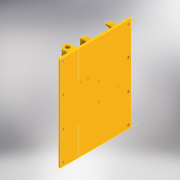
# Autodesk Inventor part: Carcasa
Saved by Autodesk Inventor 2021 (Build 250183000, 183)
## iProperties
Created: 2024-02-25
Part Number: Carcasa
Material: PLA
Document SubType Name: Modeling
Designer: Martin
Density: 1.27 g/cm^3
Appearance: PLA
Mass: 404.193 g
Surface Area: 1591.38 cm^2
Volume: 318.262 cm^3
Author: Martin
Autodesk Inventor part; units mm, degrees
ref_plane "YZ Plane" through (0, 0, 0) normal (1, 0, 0) x (0, 1, 0)
ref_plane "XZ Plane" through (0, 0, 0) normal (0, 1, 0) x (-1, 0, 0)
ref_plane "XY Plane" through (0, 0, 0) normal (0, 0, 1) x (1, 0, 0)
sketch "Sketch1" plane through (0, 0, 0) normal (0, 1, 0) x (-1, 0, 0)
  circle A0 centre (14, 22.0693) radius 4.1
  line L0 (0, 9.3293) -> (0, 34.8093) projected
  circle A1 centre (14, 22.0693) radius 9.1
  line L1 (14, 12.9693) -> (0, 12.9693)
  line L2 (14, 31.1693) -> (0, 31.1693)
  dimension "d0" = 8.2
  dimension "d7" = 14
  dimension "d20" = 5
  constraints: 4 end point, 2 centre point, 2 point on circle, 2 point on line, 1 parallel, 1 perpendicular
  measures "d0" diameter of A0
  measures "d7" distance from line of L0 A0.centre
  measures "d20" radial gap between concentric circles of A0 A1
extrude "Extrusion1" add sketch "Sketch1" along normal blind 60
sketch "Sketch3" plane through (0, 0, 0) normal (1, 0, 0) x (0, 1, 0)
  line L0 (0, 8.1261) -> (0, 35.9865) projected
  line L1 (0, 35.9865) -> (60, 35.9865) projected
  line L2 (60, 8.1261) -> (60, 35.9865) projected
  line L3 (0, 8.1261) -> (60, 8.1261) projected
  line L4 (0, 12.9691) -> (60, 12.9691)
  line L5 (60, 12.9691) -> (60, -77.0309)
  line L6 (60, -77.0309) -> (0, -77.0309)
  line L7 (8, -77.0309) -> (8, 12.9691)
  line L8 (12, -73.0309) -> (64, -73.0309)
  line L9 (56, -18.0309) -> (56, -14.0309)
  line L10 (-3, -73.0309) -> (37, -73.0309)
  line L11 (45, -75.0309) -> (45, -18.0309)
  line L12 (45, -18.0309) -> (12, -18.0309)
  line L13 (8, -14.0309) -> (49, -14.0309)
  line L14 (49.0192, -13.1359) -> (49.0192, -77.0309)
  line L15 (41.0192, -77.0309) -> (7, -77.0309)
  line L16 (8, -77.0309) -> (8, -14.0309)
  line L17 (12, -18.0309) -> (12, -24.0309)
  line L18 (12, -24.0309) -> (8, -24.0309)
  line L19 (-3, -73.0309) -> (0, -73.0309)
  line L20 (60, 17.9693) -> (0, 17.9693) projected
  line L21 (0, 12.9693) -> (60, 12.9693) projected
  line L22 (0, 12.9693) -> (0, 31.1693) projected
  line L23 (8, -73.0309) -> (12, -73.0309)
  line L24 (12, -73.0309) -> (12, -67.0309)
  line L25 (12, -67.0309) -> (8, -67.0309)
  line L26 (0, -67.0309) -> (0, -73.0309)
  line L27 (41, -14.0309) -> (0, -14.0309)
  line L28 (8, -14.0309) -> (8, -77.0309)
  line L29 (0, -77.0309) -> (41, -77.0309)
  line L30 (49, -77.0309) -> (49, -14.0309)
  line L31 (4, -73.0309) -> (37, -73.0309)
  line L32 (45, -73.0309) -> (45, -18.0309)
  line L33 (45, -18.0309) -> (12, -18.0309)
  line L34 (12, -18.0309) -> (12, -24.0309)
  line L35 (4, -67.0309) -> (4, -73.0309)
  line L36 (0, -77.0309) -> (0, 12.9691)
  line L37 (45, -75.0309) -> (12, -75.0309)
  line L38 (12, -75.0309) -> (12, -73.0309)
  line L39 (41.0192, -79.0309) -> (7, -79.0309)
  line L40 (8, -77.0309) -> (8, -79.0309)
  line L41 (41.0192, -79.0309) -> (49, -79.0309)
  line L42 (49, -79.0309) -> (49, -77.0309)
  line L43 (8, -67.0309) -> (6, -67.0309)
  line L44 (6, -67.0309) -> (6, -79.0309)
  line L45 (6, -79.0309) -> (8, -79.0309)
  line L46 (8, -14.0309) -> (6, -14.0309)
  line L47 (6, -24.0309) -> (6, -14.0309)
  line L48 (6, -24.0309) -> (8, -24.0309)
  line L49 (10, -24.0309) -> (10, -18.0309)
  line L50 (10, -18.0309) -> (12, -18.0309)
  line L51 (4, -73.0309) -> (4, -79.0309)
  line L52 (4, -79.0309) -> (6, -79.0309)
  line L53 (10, -67.0309) -> (10, -75.0309)
  line L54 (10, -75.0309) -> (12, -75.0309)
  line L55 (4, -67.0309) -> (6, -67.0309)
  line L56 (10, -75.0309) -> (8, -75.0309)
  point P0 (0, 0)
  point P1 (4, 104.056)
  point P2 (0, -73.0309)
  point P3 (49.0192, -73.0309)
  point P4 (49.0192, -77.0309)
  point P5 (8, -14.0309)
  point P6 (8, -24.0309)
  point P7 (45, -73.0309)
  point P8 (8, 8.1261)
  point P9 (0, -14.0309)
  point P10 (8, -73.0309)
  point P11 (8, -77.0309)
  point P12 (8, -67.0309)
  point P13 (12, -73.0309)
  point P14 (49, -73.0309)
  point P15 (0, -73.0309)
  point P16 (8, -77.0309)
  point P17 (6, -77.0309)
  dimension "d9" = 60
  dimension "d11" = 4
  dimension "d12" = 33
  dimension "d13" = 57
  dimension "d14" = 4
  dimension "d15" = 6
  dimension "d21" = 4
  dimension "d22" = 4
  dimension "d23" = 6
  dimension "d100" = 2
  dimension "d101" = 2
  constraints: 100 end point, 19 perpendicular, 13 parallel, 9 point on line, 8 horizontal, 5 vertical, 2 midpoint
  measures "d9" distance of L6.end L5.end
  measures "d11" distance between parallel lines of L6 L8
  measures "d12" distance of L12.end L11.end
  measures "d13" distance of L11.end L11.start
  measures "d14" distance between parallel lines of L12 L13
  measures "d15" distance of L12.end L17.end
  measures "d21" distance between parallel lines of L16 L17
  measures "d22" distance of L25.end L24.end
  measures "d23" distance of L35.end L35.start
  measures "d100" distance between parallel lines of L15 L39
  measures "d101" distance of L25.end L43.end
extrude "Extrusion2" add sketch "Sketch3" against normal blind 4 contours L0 L4 L7 L3 | L3 L7 L27 L36 | L7 L4 L2 L3 | L3 L5 L8 L30 L13 L7 | L27 L47 L48 L7 L43 L55 L35 L10 L26 L36 | L13 L30 L8 L11 L12 L50 L49 L18 L7 | L7 L48 L47 L27 | L5 L6 L14 L8 | L18 L17 L12 L11 L8 L24 L25 L7 | L10 L51 L6 L36 | L14 L6 L30 L8 | L25 L53 L10 L7 | L7 L10 L44 L43 | L49 L50 L17 L18 | L35 L55 L44 L10 | L10 L44 L6 L51 | L30 L6 L7 L56 L54 L37 L11 L8 | L10 L53 L56 L7 | L7 L6 L44 L10 | L25 L24 L10 L53 | L11 L37 L38 L8 | L10 L38 L54 L53
extrude "Extrusion3" add sketch "Sketch3" against normal blind 24 contours L13 L30 L8 L11 L12 L50 L49 L18 L7 | L7 L48 L47 L27 | L25 L53 L10 L7 | L7 L10 L44 L43 | L30 L6 L7 L56 L54 L37 L11 L8 | L10 L53 L56 L7 | L7 L6 L44 L10
sketch "Sketch5" plane through (0, 60, -77.0309) normal (0, 0, -1) x (-1, 0, 0)
  line L0 (0, -60) -> (14, -60) projected
  line L1 (14, -60) -> (14, 0) projected
  line L2 (0, 0) -> (14, 0) projected
  line L3 (0, -60) -> (0, 0) projected
  line L4 (4, -54) -> (4, -60) projected
  line L5 (0, 0) -> (4, 0) projected
  line L6 (0, -60) -> (0, 0) projected
  line L7 (0, -60) -> (4, -60) projected
  line L8 (24, -11) -> (24, -54) projected
  line L9 (0, 0) -> (4, 0)
  line L10 (4, 0) -> (4, -60)
  line L11 (4, -60) -> (0, -60)
  line L12 (0, -60) -> (0, 0)
  line L13 (4, 0) -> (4, -11) projected
  line L14 (4, -11) -> (24, -11) projected
  line L15 (4, -54) -> (24, -54) projected
  point P0 (4, -10.9808)
  constraints: 8 end point, 2 parallel, 1 horizontal, 1 perpendicular, 1 point on line
extrude "Extrusion4" add sketch "Sketch5" along normal blind 20 contours L3 L2 L10 L4 L0
sketch "Sketch6" plane through (-14, 0, 31.1693) normal (0, 0, 1) x (1, 0, 0)
  line L0 (10, 0) -> (10, 60) projected
  line L1 (0, 0) -> (14, 0) projected
  line L2 (14, 0) -> (14, 60) projected
  line L3 (0, 60) -> (14, 60) projected
  line L4 (0, 0) -> (0, 60) projected
extrude "Extrusion5" add sketch "Sketch6" along normal blind 20 contours L0 L3 L2 L1
sketch "Sketch8" plane through (-4, 0, 0) normal (-1, 0, 0) x (0, 0, 1)
  line L0 (31.1693, 0) -> (51.1693, 0) projected
  line L1 (31.1693, 0) -> (31.1693, 60) projected
  line L2 (31.1693, 0) -> (51.1693, 0) projected
  line L3 (51.1693, 60) -> (51.1693, 0) projected
  line L4 (31.1693, 60) -> (51.1693, 60) projected
  line L5 (51.1693, 60) -> (51.1693, 0) projected
  line L6 (-77.0309, 49) -> (-14.0309, 49) projected
  line L7 (-14.0309, 49) -> (-14.0309, 6) projected
  line L8 (-24.0309, 6) -> (-24.0309, 10) projected
  line L9 (-18.0309, 10) -> (-18.0309, 45) projected
  line L10 (-18.0309, 45) -> (-75.0309, 45) projected
  line L11 (-67.0309, 10) -> (-67.0309, 6) projected
  line L12 (-77.0309, 49) -> (-77.0309, 6) projected
  line L13 (12.9691, 60) -> (-97.0309, 60) projected
  line L14 (-97.0309, 0) -> (-97.0309, 60) projected
  line L15 (12.9691, 0) -> (-97.0309, 0) projected
  line L16 (12.9691, 0) -> (12.9691, 60) projected
  line L17 (-75.0309, 45) -> (-75.0309, 10) projected
  line L18 (-14.0309, 6) -> (-24.0309, 6) projected
  line L19 (-24.0309, 10) -> (-18.0309, 10) projected
  line L20 (-75.0309, 10) -> (-67.0309, 10) projected
  line L21 (-67.0309, 6) -> (-77.0309, 6) projected
  point P0 (0, 0)
  point P1 (45.1693, 8)
  point P2 (-91.0309, 8)
  point P3 (-97.0309, 90)
  dimension "d34" = 8
  dimension "d92" = 6
  dimension "d93" = 6
  dimension "d94" = 8
  measures "d34" distance from line of L0 point (45.169, 8)
  measures "d92" distance from line of L3 point (45.169, 8)
  measures "d93" distance from line of L14 point (-91.031, 8)
  measures "d94" distance from line of L15 point (-91.031, 8)
hole "Hole1" at (-4, 8, 45.1693) at (-4, 8, -91.0309) direction (1, 0, 0) diameter 4.134 depth 14.2 tip angle 118 thread size "M5x0.8" class "6H" standard "ISO Metric profile"
sketch "Sketch9" plane through (-4, 0, 0) normal (-1, 0, 0) x (0, 0, 1)
  line L0 (-84.9995, 99.1576) -> (5.0005, 99.1576)
  line L1 (5.0005, 99.1576) -> (5.0005, 60.1576)
  line L2 (5.0005, 60.1576) -> (-84.9995, 60.1576)
  line L3 (-84.9995, 60.1576) -> (-84.9995, 99.1576)
  line L4 (-80.9995, 64.1576) -> (1.0005, 64.1576)
  line L5 (1.0005, 64.1576) -> (1.0005, 99.1576)
  line L6 (-80.9995, 99.1576) -> (-80.9995, 64.1576)
  point P0 (0, 0)
  dimension "d46" = 4
  dimension "d102" = 82
  dimension "d103" = 90
  dimension "d104" = 4
  dimension "d105" = 35
  constraints: 14 end point, 3 parallel, 2 point on line, 1 horizontal, 1 perpendicular
  measures "d46" distance between parallel lines of L2 L4
  measures "d102" distance of L4.start L4.end
  measures "d103" distance of L1.end L2.end
  measures "d104" distance between parallel lines of L1 L5
  measures "d105" distance of L6.start L4.start
extrude "Extrusion7" add sketch "Sketch9" along normal blind 10 contours L0 L6 L4 L5 L1 L2 L3
sketch "Sketch10" plane through (-4, 0, 12.9691) normal (0, -1, 0) x (1, 0, 0)
  line L0 (-20, -37) -> (-20, -80) projected
  line L1 (-20, -88) -> (-20, -31) projected
  line L2 (-20, -37) -> (-20, -27) projected
  line L3 (4, 0) -> (0, 0) projected
  line L4 (0, -7.9687) -> (-10, -7.9687) projected
  line L5 (-10, -97.9687) -> (-10, -7.9687) projected
  line L6 (0, -97.9687) -> (-10, -97.9687) projected
  line L7 (-10, 18.2002) -> (0, 18.2002) projected
  arc A0 (-10, 18.2002) -> (-10, 0.0002) centre (-10, 9.1002) ccw projected
  line L8 (4, 0.0002) -> (-10, 0.0002) projected
  line L9 (4, 0.0002) -> (4, 38.2002) projected
  line L10 (0, 38.2002) -> (4, 38.2002) projected
  line L11 (0, 18.2002) -> (0, 38.2002) projected
  circle A1 centre (-10, 9.1002) radius 4.1 projected
  arc A2 (-10, 18.7002) -> (-10, -0.4998) centre (-10, 9.1002) ccw
  line L12 (-10, 18.7002) -> (-0.5, 18.7002)
  line L13 (-0.5, 18.7002) -> (-0.5, 38.2002)
  line L14 (-10.5, -7.4687) -> (0.5, -7.4687)
  line L15 (-20.5, -86) -> (-20.5, -31)
  line L16 (-20.5, -26.5) -> (-0.5, -26.5)
  line L17 (-0.5, -110) -> (-0.5, -90.5)
  line L18 (-0.5, -90.5) -> (-20.5, -90.5)
  line L19 (-20.5, -90.5) -> (-20.5, -79.5)
  line L20 (-0.5, -37.5) -> (-20.5, -37.5)
  line L21 (-20.5, -37.5) -> (-20.5, -26.5)
  line L22 (-10.5, -7.4687) -> (-10.5, -7.9687)
  line L23 (0.5, -37) -> (0.5, -37.5)
  line L24 (0.5, -80) -> (0.5, -90.2732)
  line L25 (0.5, -7.4687) -> (0.5, -7.9687)
  line L26 (0.5, -26.5) -> (0.5, -27)
  line L27 (5, -37) -> (5, -37.5)
  line L28 (5, -26.5) -> (5, -27)
  line L29 (-1, -7.9687) -> (-1, -7.4687)
  line L30 (-1, 0) -> (-1, 0.0002)
  line L31 (-0.5, -27) -> (-0.5, -0.4998)
  line L32 (-0.5, -0.4998) -> (-10, -0.4998)
  line L33 (-4.5, 26.2002) -> (-4.5, 38.2002)
  line L34 (4.5, -12.9691) -> (4.5, -8.4691)
  line L35 (4.5, -8.4691) -> (-4.5, -8.4691)
  line L36 (-0.5, -110) -> (-4.5, -110)
  line L37 (-0.5, 38.2002) -> (-4.5, 38.2002)
  line L38 (-4.5, -27) -> (-4.5, -26.5)
  line L39 (-4.5, -110) -> (-4.5, -98)
  line L40 (-4.5, -98) -> (-46.7089, -98) construction
  line L41 (-46.7089, -98) -> (-46.7089, -38.6877) construction
  line L42 (-46.7089, -38.6877) -> (-46.7089, 26.2002) construction
  line L43 (-46.7089, 26.2002) -> (-4.5, 26.2002) construction
  spline S0 degree 4 poles (-4.5, -98) (-46.7089, -98) (-46.7089, -38.6877) (-46.7089, 26.2002) (-4.5, 26.2002) knots 1 1 1 1 1 2 2 2 2 2
  line L44 (4, 0) -> (4, -110) projected
  line L45 (0, 0) -> (0, -110) projected
  line L46 (4, -110) -> (0, -110) projected
  line L47 (0, -97.9687) -> (0, -7.9687) projected
  point P0 (4, -12.9691)
  point P1 (-20, -90)
  point P2 (-20, -86)
  point P3 (-10.5, -26.5)
  point P4 (-0.5, -7.4687)
  point P5 (-0.5, -8.4691)
  point P6 (-0.5, -7.9687)
  point P7 (-2.5, 38.2002)
  point P8 (2, 38.2002)
  point P9 (-10, -26.5)
  dimension "d49" = 0.5
  dimension "d51" = 0.5
  dimension "d52" = 0.5
  dimension "d64" = 12
  dimension "d65" = 12
  constraints: 56 end point, 12 point on line, 3 midpoint, 2 horizontal, 2 parallel, 2 point on circle, 2 vertical alignment, 1 centre point, 1 horizontal alignment, 1 perpendicular, 1 vertical, 5 other
  measures "d49" radial gap between concentric circles of A0 A2
  measures "d51" distance between parallel lines of L4 L14
  measures "d52" distance between parallel lines of L1 L15
  measures "d64" distance of L36.end L39.end
  measures "d65" distance of L33.start L33.end
extrude "Extrusion8" add sketch "Sketch10" against normal blind 4 separate body contours L14 L29 L4 L5 L16 L21 L15 L19 L18 S0 L33 L37 L13 L12 A2 L32 L31 | L31 L16 L5 L4 | L17 L36 L39 S0 L6 | L6 S0 L5 L18 L17
ref_plane "Work Plane2" through (-4, 90, 12.9691) normal (0, -1, 0) x (1, 0, 0)
sketch "Sketch12" plane through (-4, 4, 12.9691) normal (0, 1, 0) x (1, 0, 0)
  spline S0 degree 4 poles (-4.5, 98) (-46.7089, 98) (-46.7089, 38.6877) (-46.7089, -26.2002) (-4.5, -26.2002) knots 0 0 0 0 0 1 1 1 1 1 projected
  line L0 (-0.5, -38.2002) -> (-0.5, -18.7002) projected
  line L1 (-0.5, 90.5) -> (-0.5, 110) projected
  line L2 (-4.5, 110) -> (-4.5, 98) projected
  line L3 (-0.5, 110) -> (-4.5, 110) projected
  line L4 (-4.5, -26.2002) -> (-4.5, -38.2002) projected
  line L5 (-4.5, -38.2002) -> (-0.5, -38.2002) projected
  line L6 (-4.5, -22.2002) -> (-0.5, -22.2002)
  line L7 (-4.5, 94) -> (-0.5, 94)
  spline S1 degree 5 poles (-4.5, 94) (-7.1215, 93.9998) (-9.7387, 93.7622) (-12.3383, 93.2317) (-17.1322, 91.5122) (-21.2907, 88.5828) (-23.0896, 86.9249) (-26.5639, 82.9724) (-29.2294, 78.4241) (-30.4611, 75.8785) (-32.7694, 70.2242) (-34.4111, 64.34) (-35.1383, 61.1404) (-36.3718, 54.4138) (-37.0751, 47.6105) (-37.3139, 44.059) (-37.5528, 36.9107) (-37.3116, 29.7623) (-37.0703, 26.1763) (-36.3594, 19.2444) (-35.1261, 12.3868) (-34.3944, 9.0916) (-32.7392, 2.9879) (-30.4285, -2.8979) (-29.1879, -5.5733) (-26.5208, -10.3549) (-23.0359, -14.5656) (-21.2378, -16.3424) (-17.1236, -19.4674) (-12.3105, -21.3549) (-9.7241, -21.9403) (-7.114, -22.1995) (-4.5, -22.2002) knots 0 0 0 0 0 0 0.088173 0.088173 0.088173 0.169677 0.169677 0.169677 0.264582 0.264582 0.264582 0.37484 0.37484 0.37484 0.494511 0.494511 0.494511 0.615347 0.615347 0.615347 0.728782 0.728782 0.728782 0.827786 0.827786 0.827786 0.912074 0.912074 0.912074 1 1 1 1 1 1
  point P0 (4, 12.9691)
  dimension "d67" = 4
  constraints: 4 end point, 2 point on line, 2 vertical alignment, 1 parallel, 1 perpendicular, 2 other
extrude "Extrusion10" add sketch "Sketch12" along normal up to surface (86 mm away) bodies 2
sketch "Sketch13" plane through (-8.5, 4, 39.1693) normal (-1, 0, 0) x (0, 0, 1)
  circle A0 centre (6, 4) radius 2.067 projected
  circle A1 centre (6, 59) radius 2.067 projected
  circle A2 centre (-130.2002, 4) radius 2.067 projected
  circle A3 centre (-130.2002, 59) radius 2.067 projected
  point P0 (-39.1693, -4)
hole "Hole2" at (-8.5, 8, -91.0309) at (-8.5, 63, -91.0309) at (-8.5, 8, 45.1693) at (-8.5, 63, 45.1693) direction (1, 0, 0) diameter 4.134 depth 14.2 tip angle 118 bodies 2 thread size "M5x0.8" class "6H" standard "ISO Metric profile"
mirror "Mirror2" about plane through (-27.6044, 90, -22.9308) normal (0, 1, 0) of "Extrusion8", "Extrusion10", "Hole2" bodies 2
sketch "Sketch18" plane through (0, 60, 0) normal (0, 1, 0) x (1, 0, 0)
  line L0 (-4, -12.9691) -> (-4, 97.0309) projected
  line L1 (0, -51.1693) -> (-4, -51.1693)
  line L2 (-4, -51.1693) -> (-4, 97.0309)
  line L3 (-4, 97.0309) -> (0, 97.0309)
  line L4 (0, 97.0309) -> (0, -51.1693)
  point P0 (0, 0)
  constraints: 8 end point, 2 parallel, 1 horizontal, 1 perpendicular
extrude "Extrusion15" add sketch "Sketch18" along normal up to surface (39.1576 mm away) bodies 1
pattern_linear "Rectangular Pattern2" count 2 spacing 60 along (0, 1, 0) of "Hole1" bodies 1
sketch "Sketch19" plane through (0, 60, 0) normal (0, 1, 0) x (1, 0, 0)
  circle A0 centre (-14, -22.0693) radius 4.1 projected
  line L0 (-4, -31.1693) -> (-4, -12.9693) projected
  line L1 (-4, -12.9693) -> (-14, -12.9693) projected
  arc A1 (-14, -12.9693) -> (-14, -31.1693) centre (-14, -22.0693) ccw projected
  line L2 (-14, -31.1693) -> (-4, -31.1693) projected
  point P0 (0, 0)
extrude "Extrusion16" cut sketch "Sketch19" against normal blind 15 bodies 1
mirror "Mirror5" about plane through (-4, 99.1576, 5.0005) normal (0, 1, 0) of "Extrusion3", "Extrusion2", "Hole1", "Rectangular Pattern2", "Extrusion7", "Extrusion15", "Extrusion5", "Extrusion4", "Extrusion16", "Extrusion1" bodies 1
sketch "Sketch20" plane through (-4, 64.1576, -80.9995) normal (-1, 0, 0) x (0, 0, 1)
  point P0 (80.9995, -64.1576)
  point P1 (13.533, 23.3339)
  point P2 (52.0117, 16.488)
  point P3 (52.0117, 54.7306)
hole "Hole3" at (-4, 87.4915, -67.4665) at (-4, 80.6456, -28.9879) at (-4, 118.8881, -28.9879) direction (1, 0, 0) diameter 3 depth 14.2 tip angle 118 bodies 1
sketch "Sketch21" plane through (-4, 0, 0) normal (-1, 0, 0) x (0, 0, 1)
  point P0 (0, 0)
sketch "Sketch22" plane through (-14, 60.1576, 5.0005) normal (0, 0, 1) x (1, 0, 0)
  line L0 (10, 0) -> (10, 78) projected
  line L1 (10, 78) -> (0, 78) projected
  line L2 (0, 0) -> (0, 78) projected
  line L3 (10, 0) -> (0, 0) projected
  point P0 (14, -60.1576)
extrude "Extrusion17" cut sketch "Sketch22" against normal up to surface (90 mm away) bodies 1
sketch "Sketch23" plane through (-4, 0, 0) normal (-1, 0, 0) x (0, 0, 1)
  line L0 (-13.2015, 56.3542) -> (-83.2015, 56.3542)
  line L1 (-83.2015, 56.3542) -> (-83.2015, 138.3542)
  line L2 (-83.2015, 138.3542) -> (-13.2015, 138.3542)
  line L3 (-13.2015, 138.3542) -> (-13.2015, 56.3542)
  line L4 (-81.206, 110.8556) -> (-81.206, 137.4428) construction
  line L5 (-81.206, 137.4428) -> (-78.0296, 137.4428) construction
  line L6 (-78.0296, 137.4428) -> (-78.0296, 110.8556) construction
  line L7 (-78.0296, 110.8556) -> (-81.206, 110.8556) construction
  point P0 (0, 0)
  constraints: 8 end point, 2 parallel, 1 horizontal, 1 perpendicular, 2 other
sketch "Sketch24" plane through (-4, 0, 0) normal (-1, 0, 0) x (0, 0, 1)
  line L0 (-10.7811, 56.3724) -> (21.2189, 56.3724)
  line L1 (21.2189, 56.3724) -> (21.2189, 98.3724)
  line L2 (21.2189, 98.3724) -> (-10.7811, 98.3724)
  line L3 (-10.7811, 98.3724) -> (-10.7811, 56.3724)
  line L4 (-8.7811, 96.3724) -> (19.2189, 96.3724)
  line L5 (19.2189, 96.3724) -> (19.2189, 58.3724)
  line L6 (19.2189, 58.3724) -> (-8.7811, 58.3724)
  line L7 (-8.7811, 58.3724) -> (-8.7811, 96.3724)
  line L8 (16.2649, 96.3724) -> (16.2649, 98.3724)
  line L9 (-5.6057, 96.3724) -> (-5.6057, 98.3724)
  point P0 (0, 0)
  dimension "d117" = 32
  dimension "d118" = 42
  dimension "d119" = 2
  constraints: 20 end point, 5 parallel, 4 point on line, 3 perpendicular, 1 horizontal, 3 other
  measures "d117" distance of L2.end L1.end
  measures "d118" distance of L1.end L0.end
  measures "d119" distance between parallel lines of L2 L4
extrude "Extrusion18" add sketch "Sketch24" along normal blind 10 contours L3 L2 L9 L4 L7 L6 L5 L8 L1 L0 bodies 1
sketch "Sketch25" plane through (-4, 0, 0) normal (-1, 0, 0) x (0, 0, 1)
  line L0 (-10.7233, 138.2024) -> (14.7767, 138.2024)
  line L1 (14.7767, 138.2024) -> (14.7767, 123.0024)
  line L2 (14.7767, 123.0024) -> (-10.7233, 123.0024)
  line L3 (-10.7233, 123.0024) -> (-10.7233, 138.2024)
  line L4 (-9.9955, 127.3092) -> (8.9668, 127.3092) construction
  line L5 (8.9668, 127.3092) -> (8.9668, 124.1353) construction
  line L6 (8.9668, 124.1353) -> (-9.9955, 124.1353) construction
  line L7 (-9.9955, 124.1353) -> (-9.9955, 127.3092) construction
  line L8 (-7.0549, 59.6709) -> (-7.0549, 76.9684) construction
  line L9 (-7.0549, 76.9684) -> (-4.0069, 76.9684) construction
  line L10 (-4.0069, 76.9684) -> (-4.0069, 59.6709) construction
  line L11 (-4.0069, 59.6709) -> (-7.0549, 59.6709) construction
  line L12 (-73.5211, 12.3758) -> (-73.5211, 39.3435) construction
  line L13 (-73.5211, 39.3435) -> (-70.3446, 39.3435) construction
  line L14 (-70.3446, 39.3435) -> (-70.3446, 12.3758) construction
  line L15 (-70.3446, 12.3758) -> (-73.5211, 12.3758) construction
  point P0 (0, 0)
  constraints: 8 end point, 2 parallel, 1 horizontal, 1 perpendicular, 6 other
sketch "Sketch26" plane through (-4, 0, 0) normal (-1, 0, 0) x (0, 0, 1)
  point P0 (0, 0)
  point P1 (9.6155, 135.1004)
  point P2 (-6.0605, 135.1004)
hole "Hole4" at (-4, 135.1004, 9.6155) at (-4, 135.1004, -6.0605) direction (1, 0, 0) diameter 3 depth 14.2 tip angle 118 bodies 1
body "Solid1"
body "Solid2"
